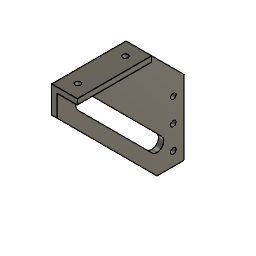
DockingMechanismBracketL (Autodesk Fusion 360 design; units mm, degrees)
Autodesk Fusion 360 part; units mm, degrees
sketch "Sketch4" plane through (0, 0, 0) normal (1, 0, 0) x (0, 1, 0)
  line L0 (-93.8909, 93.8909) -> (-38.8909, 93.8909)
  line L1 (-38.8909, 93.8909) -> (0, 55)
  line L2 (0, 55) -> (0, 0)
  line L3 (0, 0) -> (-20, 0)
  line L4 (-93.8909, 93.8909) -> (-93.8909, 73.8909)
  line L5 (-93.8909, 73.8909) -> (-20, 0)
  line L6 (-16.4645, 23.5355) -> (-71.4645, 78.5355)
  arc A0 (-71.4645, 78.5355) -> (-78.5355, 71.4645) centre (-75, 75) ccw
  line L7 (-78.5355, 71.4645) -> (-23.5355, 16.4645)
  arc A1 (-23.5355, 16.4645) -> (-16.4645, 23.5355) centre (-20, 20) ccw
  line L8 (-20, 20) -> (-75, 75) construction
  circle A2 centre (-8, 10) radius 2
  circle A3 centre (-8, 45) radius 2
  line L9 (-8, 45) -> (-8, 10) construction
  line L10 (0, 27.5) -> (-8, 27.5) construction
  circle A4 centre (-8, 27.5) radius 2
  dimension "d15" = 55
  dimension "d16" = 135
  dimension "d17" = 55
  dimension "d18" = 55
  dimension "d19" = 20
  dimension "d20" = 20
  dimension "d21" = 10
  dimension "d22" = 4
  dimension "d23" = 4
  dimension "d24" = 8
  dimension "d25" = 35
  dimension "d35" = 4
  constraint horizontal L0
  constraint vertical L2
  constraint perpendicular L2 L3
  constraint vertical L4
  constraint tangent L6 A0
  constraint tangent A0 L7
  constraint parallel L6 L7
  constraint tangent L7 A1
  constraint tangent L6 A1
  constraint coincident A3.centre L9.start
  constraint coincident A2.centre L9.end
  constraint vertical L9
  constraint midpoint L2 L10.start
  constraint midpoint L9 L10.end
  constraint perpendicular L2 L10
  constraint coincident L0.start L4.start
  constraint coincident L2.end L3.start
  constraint coincident L10.end A4.centre
  measures "d15" distance of L0.start L0.end
  measures "d16" angle of L0 L1
  measures "d17" distance of L0.end L1.end
  measures "d18" distance of L1.end L2.end
  measures "d19" distance of L2.end L3.end
  measures "d20" distance of L0.start L4.end
  measures "d21" diameter of A0
  measures "d22" diameter of A2
  measures "d23" diameter of A3
  measures "d24" distance of L2 L9
  measures "d25" distance of A3.centre A2.centre
  measures "d35" diameter of A4
extrude "Extrude1" add sketch "Sketch4" along normal blind 4
sketch "Sketch5" plane through (0, 0, 93.8909) normal (0, 0, 1) x (-1, 0, 0)
  line L0 (0, 38.8909) -> (0, 93.8909)
  line L1 (0, 93.8909) -> (-4, 93.8909)
  line L2 (-4, 93.8909) -> (-4, 38.8909)
  line L3 (-4, 38.8909) -> (0, 38.8909)
  line L4 (0, 93.8909) -> (-19, 93.8909)
  line L5 (-19, 93.8909) -> (-19, 38.8909)
  line L6 (-19, 38.8909) -> (0, 38.8909)
  line L7 (0, 38.8909) -> (0, 93.8909)
  circle A0 centre (-9.5, 83.8909) radius 2
  circle A1 centre (-9.5, 48.8909) radius 2
  line L8 (-9.5, 83.8909) -> (-9.5, 48.8909) construction
  line L9 (-9.5, 66.3909) -> (0, 66.3909) construction
  line L10 (-9.5, 48.8909) -> (-9.5, 38.8909) construction
  dimension "d28" = 55
  dimension "d30" = 4
  dimension "d31" = 4
  dimension "d32" = 35
  dimension "d36" = 19
  constraint horizontal L4
  constraint vertical L5
  constraint horizontal L6
  constraint vertical L7
  constraint coincident L0.end L1.start
  constraint coincident A0.centre L8.start
  constraint coincident A1.centre L8.end
  constraint midpoint L8 L9.start
  constraint midpoint L7 L9.end
  constraint perpendicular L7 L9
  constraint midpoint L6 L10.end
  constraint perpendicular L6 L10
  constraint vertical L8
  measures "d28" distance of L0.end L0.start
  measures "d30" diameter of A0
  measures "d31" diameter of A1
  measures "d32" vertical distance of A0.centre A1.centre
  measures "d36" distance of L0.end L4.end
extrude "Extrude3" add sketch "Sketch5" against normal blind 4 contours L2 L4 L5 L6
